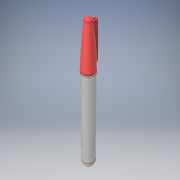
# Autodesk Inventor part: Pen_Sharpie
Saved by Autodesk Inventor 2019 (Build 230136000, 136)
## iProperties
Created: 2021-01-19
Part Number: Pen_Sharpie
Material: ABS Plastic
Document SubType Name: Modeling
Designer: zhanb
Density: 1.06 g/cm^3
Appearance: Smooth - White
Author: zhanb
Autodesk Inventor part; units mm, degrees
ref_plane "YZ Plane" through (0, 0, 0) normal (1, 0, 0) x (0, 1, 0)
ref_plane "XZ Plane" through (0, 0, 0) normal (0, 1, 0) x (-1, 0, 0)
ref_plane "XY Plane" through (0, 0, 0) normal (0, 0, 1) x (1, 0, 0)
sketch "Sketch1" plane through (0, 0, 0) normal (1, 0, 0) x (0, 1, 0)
  line L0 (-68.58, 6.096) -> (17.78, 6.096) construction
  line L1 (68.58, 6.096) -> (68.58, -6.096) construction
  line L2 (68.58, -6.096) -> (17.78, -6.096) construction
  line L3 (-68.58, -6.096) -> (-68.58, -1.7607) construction
  line L4 (-68.58, 6.096) -> (68.58, -6.096) construction
  line L5 (68.58, 6.096) -> (-68.58, -6.096) construction
  line L6 (17.78, -6.096) -> (17.78, 6.096) construction
  line L7 (17.78, -6.096) -> (-68.58, -6.096) construction
  line L8 (17.78, 6.096) -> (68.58, 6.096) construction
  arc A0 (19.05, -6.4135) -> (65.4643, -3.5286) centre (19.05, 368.4065) ccw
  arc A1 (65.4643, -3.5286) -> (68.58, 0) centre (65.024, 0) ccw
  line L9 (19.05, -6.4135) -> (18.0975, -5.461)
  line L10 (18.0975, -5.461) -> (17.4625, -5.461)
  line L11 (17.4625, -5.461) -> (16.8275, -6.096)
  line L12 (16.8275, -6.096) -> (-62.8846, -5.3721)
  arc A2 (-69.215, 1.016) -> (-68.58, -1.7607) centre (-62.8266, 1.016) ccw construction
  arc A3 (-68.58, -1.7607) -> (-62.8846, -5.3721) centre (-62.8266, 1.016) ccw
  line L13 (-68.58, -1.7607) -> (-68.58, 0)
  line L14 (-68.58, 0) -> (68.58, 0)
  line L15 (-68.58, 0) -> (-68.58, 6.096) construction
  line L16 (68.58, -6.4135) -> (17.78, -6.4135) construction
  point P0 (0, 0)
  point P1 (0, 0)
  point P2 (17.78, -5.461)
  point P3 (17.78, 0)
  dimension "d0" = 12.192
  dimension "d1" = 137.16
  dimension "d3" = 50.8
  dimension "d4" = 3.556
  dimension "d5" = 0.635
  dimension "d6" = 45
  dimension "d7" = 45
  dimension "d8" = 0.635
  dimension "d9" = 0.635
  dimension "d10" = 1.016
  dimension "d11" = 5.3721
  dimension "d14" = 0.3175
  constraints: 34 end point, 8 point on circle, 7 parallel, 5 tangent, 4 centre point, 4 horizontal, 4 midpoint, 4 perpendicular, 3 point on line, 2 vertical alignment, 1 coincident, 1 horizontal alignment, 1 vertical
  measures "d0" distance of L1.start L1.end
  measures "d1" distance of L1.end L3.start
  measures "d3" distance between parallel lines of L1 L6
  measures "d4" radius of A1
  measures "d5" distance between parallel lines of L7 L10
  measures "d6" angle of L10 L9
  measures "d7" angle of L11 L10
  measures "d8" distance of L9.end L10.end
  measures "d9" distance from line of L3 A2.start
  measures "d10" distance from line of L14 A2.centre
  measures "d11" distance from line of L14 L12.end
  measures "d14" distance between parallel lines of L2 L16
revolve "Revolution1" add sketch "Sketch1" angle 360 about axis through (0, -68.58, 0) along (0, 1, 0)
sketch "Sketch2" plane through (0, 0, 0) normal (1, 0, 0) x (0, 1, 0)
  line L0 (64.008, -3.048) -> (64.008, -5.715)
  arc A0 (60.198, -9.525) -> (64.008, -5.715) centre (60.198, -5.715) ccw
  line L1 (60.198, -9.525) -> (23.368, -9.525)
  line L2 (28.7953, -7.62) -> (60.198, -7.62)
  arc A1 (60.198, -7.62) -> (62.103, -5.715) centre (60.198, -5.715) ccw
  line L3 (62.103, -5.715) -> (62.103, -3.048)
  line L4 (62.103, -3.048) -> (64.008, -3.048)
  arc A2 (28.7953, -7.62) -> (23.368, -9.525) centre (26.416, -9.525) ccw
  line L5 (-13.716, 0) -> (82.296, 0) construction
  arc A3 (65.4643, -3.5286) -> (65.4643, 3.5286) centre (65.024, 0) ccw construction
  line L6 (60.198, -7.62) -> (60.198, -3.048)
  line L7 (62.103, -3.048) -> (60.198, -3.048)
  point P0 (0, 0)
  dimension "d15" = 3.048
  dimension "d16" = 1.905
  dimension "d17" = 3.048
  dimension "d18" = 1.016
  dimension "d19" = 3.81
  dimension "d20" = 40.64
  dimension "d21" = 9.525
  constraints: 14 end point, 6 point on circle, 4 tangent, 3 centre point, 3 perpendicular, 2 vertical, 1 concentric, 1 horizontal, 1 parallel, 1 point on line
  measures "d15" radius of A2
  measures "d16" distance of L3.end L0.start
  measures "d17" distance between parallel lines of L4 L5
  measures "d18" horizontal distance of L0.start A3.centre
  measures "d19" radius of A0
  measures "d20" distance from line of L0 L1.end
  measures "d21" distance between parallel lines of L5 L1
extrude "Extrusion1" add sketch "Sketch2" along normal mid plane 3.556 contours L0 A0 L1 A2 L2 A1 L3 L4
extrude "Extrusion2" add sketch "Sketch2" along normal mid plane 1.524 contours L3 A1 L6 L7
chamfer "Chamfer1" distance 1.524 angle 45 6 edges at (1.778, 41.783, -9.525) (1.778, 62.8921, -8.4091) (1.778, 64.008, -4.4842) (-1.778, 41.783, -9.525) (-1.778, 62.8921, -8.4091) (-1.778, 64.008, -4.4842)
fillet "Fillet1" radius 0.508 3 edges at (-1.0429, 23.4719, -8.7361) (1.0429, 23.4719, -8.7361) (0, 28.7953, -7.62)
body "Solid1"
